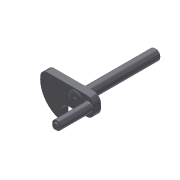
# Autodesk Inventor part: Crankshaft
Saved by Autodesk Inventor 2022 Beta2 (Build 260130000, 130) ContinuousBuild 0
## iProperties
Shininess: 64.0
Angle Display Precision: 2
Document Length Units: 11272
Document Angle Units: 11279
Document Time Units: 11290
Document Mass Units: 11286
Document Length Units Precision: 3
Document Angle Units Precision: 2
Created: 2002-04-17
Part Number: Crankshaft
Material: Steel, High Strength Low Alloy
Document SubType Name: Modeling
Designer: Nino
Density: 7.84 g/cm^3
Mass: 6068.09 g
Surface Area: 892.226 cm^2
Volume: 773.991 cm^3
Appearance: Metal-Steel (Polished)
Density: 0.0
Volumn: 0.0
Area: 0.0
PropertySet Name: Model Information
Control State: 0
Master: False
Checked Out: False
Author: Nino
Autodesk Inventor part; units mm, degrees
ref_plane "YZ Plane" through (0, 0, 0) normal (1, 0, 0) x (0, 1, 0)
ref_plane "XZ Plane" through (0, 0, 0) normal (0, 1, 0) x (-1, 0, 0)
ref_plane "XY Plane" through (0, 0, 0) normal (0, 0, 1) x (1, 0, 0)
sketch "Sketch1" plane through (0, 0, 0) normal (0, 0, 1) x (1, 0, 0)
  circle A0 centre (0, 0) radius 19.05
  circle A1 centre (0, 0) radius 28.702
  dimension "d1" = 9.652
  dimension "d38" = 38.1
  constraints: 2 centre point, 1 concentric, 1 other
  measures "d1" radial gap between concentric circles of A1 A0
  measures "d38" diameter of A0
extrude "Extrusion1" add sketch "Sketch1" against normal blind 254 contours A0
extrude "Extrusion2" add sketch "Sketch1" along normal blind 6.35 contours A0 | A1
chamfer "Chamfer1" distance 3.175 angle 45 1 edges at (-19.05, 0, -254)
sketch "Sketch2" plane through (0, 0, 6.35) normal (0, 0, 1) x (1, 0, 0)
  circle A0 centre (0, 0) radius 28.702 projected
  circle A1 centre (0, 0) radius 33.7566
  arc A2 (-68.8892, 89.446) -> (-67.2009, -88.2638) centre (-33.7441, 0.9169) ccw
  line L0 (-53.7761, -78.8636) -> (-67.2009, -88.2638)
  line L1 (0, -33.7566) -> (0, 33.7566)
  line L2 (-53.7761, 78.8636) -> (-53.7761, -78.8636)
  line L3 (-53.7761, 78.8636) -> (-68.8892, 89.446)
  line L4 (63.5, 33.7566) -> (-53.7761, 33.7566)
  line L5 (0, 0) -> (-53.7761, 0)
  line L6 (-146.05, 0) -> (-154.4505, 0)
  line L7 (63.5, -33.7566) -> (-53.7761, -33.7566)
  line L8 (0, 0) -> (63.5, 0)
  line L9 (63.5, 0) -> (63.5, -33.7566)
  line L10 (63.5, 0) -> (63.5, 33.7566)
  line L11 (-53.7761, 33.7566) -> (-123.154, 33.7566)
  line L12 (-53.7761, 0) -> (-128.9897, 0)
  line L13 (-53.7761, -33.7566) -> (-122.4589, -33.7566)
  dimension "d8" = 125
  dimension "d10" = 190.5
  dimension "d17" = 63.5
  constraints: 28 end point, 8 point on circle, 6 perpendicular, 4 horizontal, 4 point on line, 2 centre point, 2 midpoint, 2 parallel, 2 tangent, 1 collinear
  measures "d8" angle of L0 L1
  measures "d10" diameter of A2
  measures "d17" distance from line of L5.start L10
extrude "Extrusion10" add sketch "Sketch2" along normal blind 25.4 contours L8 L1 A0 | L8 A1 L1 A0 | A0 L1 L8 | A0 L1 A1 L8 | L1 L5 A0 | A0 L5 A1 L1 | L1 A1 L5 A0 | A0 L5 L1 | L8 L9 L7 A1 | A1 L4 L10 L8 | A1 L5 L2 L4 | L7 L2 L5 A1 | L2 L12 A2 L11 | L13 A2 L12 L2 | L2 L0 A2 L13
fillet "Fillet1" radius 25.4 4 edges at (-53.7761, -33.7566, 19.05) (63.5, -33.7566, 19.05) (63.5, 33.7566, 19.05) (-123.154, 33.7566, 19.05)
sketch "Sketch3" plane through (0, 0, 31.75) normal (0, 0, 1) x (1, 0, 0)
  circle A0 centre (0, 0) radius 28.702
  circle A1 centre (0, 0) radius 8.5985
  arc A2 (-103.1968, 33.7566) -> (-128.4523, 11.0619) centre (-103.1968, 8.3566) ccw projected
  arc A3 (-128.4523, 11.0619) -> (-67.2009, -88.2638) centre (-33.7441, 0.9169) ccw projected
  line L0 (-53.7761, -78.8636) -> (-67.2009, -88.2638) projected
  line L1 (-53.7761, -59.1566) -> (-53.7761, -78.8636) projected
  arc A4 (-28.3761, -33.7566) -> (-53.7761, -59.1566) centre (-28.3761, -59.1566) ccw projected
  line L2 (38.1, -33.7566) -> (-28.3761, -33.7566) projected
  arc A5 (38.1, -33.7566) -> (63.5, -8.3566) centre (38.1, -8.3566) ccw projected
  line L3 (63.5, 8.3566) -> (63.5, -8.3566) projected
  arc A6 (63.5, 8.3566) -> (38.1, 33.7566) centre (38.1, 8.3566) ccw projected
  line L4 (-103.1968, 33.7566) -> (38.1, 33.7566) projected
  constraints: 2 centre point
extrude "Extrusion5" add sketch "Sketch3" along normal blind 3.175 contours A0 | A1
extrude "Extrusion6" add sketch "Sketch3" along normal blind 6.35 contours A1
fillet "Fillet2" radius 25.4 1 edges at (-28.702, 0, 34.925)
sketch "Sketch4" plane through (0, 0, 31.75) normal (0, 0, 1) x (1, 0, 0)
  line L0 (63.5, 8.3566) -> (63.5, -8.3566)
  circle A0 centre (44.45, 0) radius 15.875
  circle A1 centre (44.45, 0) radius 9.525
  arc A2 (-28.702, 0) -> (28.702, 0) centre (0, 0) ccw projected
  arc A3 (28.702, 0) -> (-28.702, 0) centre (0, 0) ccw projected
  arc A4 (-103.1968, 33.7566) -> (-128.4523, 11.0619) centre (-103.1968, 8.3566) ccw projected
  arc A5 (-128.4523, 11.0619) -> (-67.2009, -88.2638) centre (-33.7441, 0.9169) ccw projected
  line L1 (-53.7761, -78.8636) -> (-67.2009, -88.2638) projected
  line L2 (-53.7761, -59.1566) -> (-53.7761, -78.8636) projected
  arc A6 (-28.3761, -33.7566) -> (-53.7761, -59.1566) centre (-28.3761, -59.1566) ccw projected
  line L3 (38.1, -33.7566) -> (-28.3761, -33.7566) projected
  arc A7 (38.1, -33.7566) -> (63.5, -8.3566) centre (38.1, -8.3566) ccw projected
  line L4 (63.5, 8.3566) -> (63.5, -8.3566) projected
  arc A8 (63.5, 8.3566) -> (38.1, 33.7566) centre (38.1, 8.3566) ccw projected
  line L5 (-103.1968, 33.7566) -> (38.1, 33.7566) projected
  dimension "d24" = 19.05
  dimension "d25" = 31.75
  dimension "d26" = 19.05
  constraints: 2 centre point, 2 end point
  measures "d24" distance from line of L0 A0.centre
  measures "d25" diameter of A0
  measures "d26" diameter of A1
extrude "Extrusion7" add sketch "Sketch4" along normal blind 120.65 contours A1
extrude "Extrusion8" add sketch "Sketch4" along normal blind 114.3 contours A0 A2 A3 | A3 A2 A0 picked at (58.0643, -1.2262) picked at (28.6234, 0)
fillet "Fillet3" radius 3.175 2 edges at (45.2559, 15.8545, 31.75) (45.2559, -15.8545, 31.75)
sketch "Sketch5" plane through (0, 0, -254) normal (0, 0, -1) x (-1, 0, 0)
  circle A0 centre (0, 0) radius 15.875 projected
  line L0 (6.35, 5.9176) -> (31.75, 5.9176)
  line L1 (31.75, 5.9176) -> (31.75, -6.7824)
  line L2 (31.75, -6.7824) -> (6.35, -6.7824)
  line L3 (6.35, -6.7824) -> (6.35, 5.9176)
  dimension "d32" = 12.7
  dimension "d33" = 25.4
  dimension "d34" = 6.35
  constraints: 8 end point, 2 parallel, 1 horizontal, 1 perpendicular
  measures "d32" distance of L0.end L1.end
  measures "d33" distance of L0.start L0.end
  measures "d34" distance from line of L3 A0.centre
extrude "Extrusion9" cut sketch "Sketch5" against normal blind 76.2 contours A0 L2 L3 L0 | A0 L0 L1 L2 picked at (9.525, -0.2883)
fillet "Fillet4" radius 3.175 2 edges at (-12.0759, -6.7824, -177.8) (-12.2288, 5.9176, -177.8)
equation "\"d9\" = d8"
equation "\"d12\" = d11"
equation "\"d11\" = 31.75"
body "Solid1"
